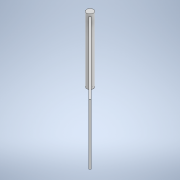
# Autodesk Inventor part: вал
Saved by Autodesk Inventor 2021 (Build 250183000, 183)
## iProperties
Created: 2023-02-16
Part Number: вал
Material: Типовые
Document SubType Name: Modeling
Designer: Tasya
Density: 1 g/cm^3
Appearance: По умолчанию
Author: Tasya
Autodesk Inventor part; units mm, degrees
ref_plane "XZ Plane" through (0, 0, 0) normal (0, 1, 0) x (-1, 0, 0)
sketch "Эскиз1" plane through (0, 0, 0) normal (0, 1, 0) x (-1, 0, 0)
  circle A0 centre (0, 0) radius 10
  dimension "d0" = 20
  constraints: 1 centre point, 1 coincident
  measures "d0" diameter of A0
extrude "Выдавливание1" add sketch "Эскиз1" along normal blind 194.4
sketch "Эскиз2" plane through (0, 0, 0) normal (0, -1, 0) x (1, 0, 0)
  circle A0 centre (0, 0) radius 7.5 construction
  point P0 (0, 7.5)
  dimension "d3" = 15
  constraints: 1 coincident, 1 vertical alignment, 2 other
hole "Отверстие1" at (0, 0, 7.5) direction (0, 1, 0) diameter 3.9 depth 6 countersink diameter 4.5 countersink angle 90
pattern_circular "Круговой массив1" count 4 over 360 about axis through (0, 0, 0) along (0, 1, 0) of "Отверстие1"
ref_plane "РабПлоскость1" through (0, 0, 0) normal (0.7071, 0, -0.7071) x (0, 1, 0)
sketch "Эскиз3" plane through (0, 0, 0) normal (0.7071, 0, -0.7071) x (0, 1, 0)
  line L0 (0, 10) -> (194.4, 10) projected
  point P0 (0, 0)
ref_plane "РабПлоскость2" through (7.0711, 0, 7.0711) normal (0.7071, 0, 0.7071) x (0, 1, 0)
sketch "Эскиз4" plane through (7.0711, 0, 7.0711) normal (0.7071, 0, 0.7071) x (0, 1, 0)
  line L0 (6, 3.3533) -> (0.3, 3.3533) projected
  line L1 (6, 7.2533) -> (0.3, 7.2533) projected
  line L2 (6, 7.2533) -> (6, 3.3533) projected
  line L3 (6, -7.2533) -> (0.3, -7.2533) projected
  line L4 (6, -3.3533) -> (0.3, -3.3533) projected
  line L5 (6, -3.3533) -> (6, -7.2533) projected
  line L6 (7, 2.5) -> (187.4, 2.5)
  line L7 (187.4, 2.5) -> (187.4, -2.5)
  line L8 (187.4, -2.5) -> (7, -2.5)
  line L9 (7, -2.5) -> (7, 2.5)
  line L10 (0, 0) -> (8, 0) construction
  line L11 (194.4, -10) -> (194.4, 10) construction
  dimension "d14" = 5
  dimension "d15" = 7
  dimension "d16" = 7
  constraints: 10 end point, 2 horizontal, 2 parallel, 1 perpendicular, 1 other
  measures "d14" distance between parallel lines of L8 L6
  measures "d15" horizontal distance of L8.end L10.start
  measures "d16" distance between parallel lines of L11 L7
extrude "Выдавливание2" add sketch "Эскиз4" along normal blind 300 and the other way blind 10
